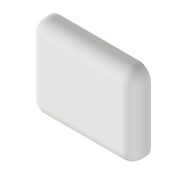
# Autodesk Inventor part: Adaptive Lid
Saved by Autodesk Inventor 2020.1 (Build 241239000, 239)
## iProperties
Created: 2019-09-12
Part Number: Adaptive Lid
Material: Generic
Document SubType Name: Modeling
Designer: thom_tremblay
Density: 1 g/cm^3
Appearance: Default
Author: thom_tremblay
Autodesk Inventor part; units mm, degrees
ref_plane "YZ Plane" through (0, 0, 0) normal (1, 0, 0) x (0, 1, 0)
ref_plane "XZ Plane" through (0, 0, 0) normal (0, 1, 0) x (-1, 0, 0)
ref_plane "XY Plane" through (0, 0, 0) normal (0, 0, 1) x (1, 0, 0)
sketch "Sketch1" plane through (0, 0, 0) normal (0, 0, 1) x (1, 0, 0)
  line L0 (-21.5469, -17.0285) -> (21.5469, -17.0285)
  line L1 (21.5469, -17.0285) -> (21.5469, 17.0285)
  line L2 (21.5469, 17.0285) -> (-21.5469, 17.0285)
  line L3 (-21.5469, 17.0285) -> (-21.5469, -17.0285)
  constraints: 8 end point, 2 parallel, 1 horizontal, 1 perpendicular
extrude "Extrusion1" add sketch "Sketch1" along normal blind 7.62
fillet "Fillet1" radius 5.08 8 edges at (-21.5469, -17.0285, 3.81) (-21.5469, 0, 7.62) (-21.5469, 17.0285, 3.81) (21.5469, 17.0285, 3.81) (21.5469, -17.0285, 3.81) (0, -17.0285, 7.62) (21.5469, 0, 7.62) (0, 17.0285, 7.62)
shell "Shell1" thickness 2.54 removed faces 1 at (5.489, -5.6762, 0)
body "Solid1"
